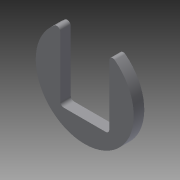
# Autodesk Inventor part: PolyfuseAdapter2
Saved by Autodesk Inventor 2015 (Build 190159000, 159)
## iProperties
Created: 2014-05-07
Part Number: PolyfuseAdapter2
Material: Generic
Document SubType Name: Modeling
Designer: STACKPOLE
Density: 1 g/cm^3
Appearance: Default
Author: STACKPOLE
Autodesk Inventor part; units mm, degrees
ref_plane "YZ Plane" through (0, 0, 0) normal (1, 0, 0) x (0, 1, 0)
ref_plane "XZ Plane" through (0, 0, 0) normal (0, 1, 0) x (-1, 0, 0)
ref_plane "XY Plane" through (0, 0, 0) normal (0, 0, 1) x (1, 0, 0)
sketch "Sketch1" plane through (0, 0, 0) normal (0, 1, 0) x (-1, 0, 0)
  arc A0 (-8.6154, 11.0352) -> (8.6154, 11.0352) centre (0, 0) ccw
  line L0 (7, 10.247) -> (7, -7)
  line L1 (6, -8) -> (-6, -8)
  line L2 (-7, -7) -> (-7, 10.247)
  arc A1 (-7, 10.247) -> (-8.6154, 11.0352) centre (-8, 10.247) ccw
  arc A2 (8.6154, 11.0352) -> (7, 10.247) centre (8, 10.247) ccw
  arc A3 (6, -8) -> (7, -7) centre (6, -7) ccw
  arc A4 (-7, -7) -> (-6, -8) centre (-6, -7) ccw
  point P0 (-7, 12.1244)
  point P1 (7, 12.1244)
  dimension "d0" = 28
  dimension "d2" = 14
  dimension "d4" = 1
  dimension "d5" = 8
  constraints: 12 point on circle, 8 tangent, 6 end point, 5 centre point, 3 equal radius, 2 point on line, 1 coincident, 1 parallel
  measures "d0" diameter of A0
  measures "d2" distance of point (-7, 12.124) point (7, 12.124)
  measures "d4" radius of A1
  measures "d5" distance from line of point (0, 0) L1
extrude "Extrusion1" add sketch "Sketch1" along normal blind 3
body "Solid1"
